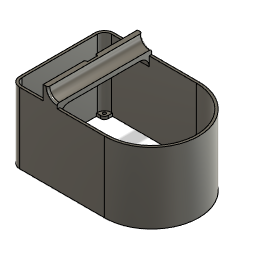
planter base v6 (Autodesk Fusion 360 design; units mm, degrees)
Autodesk Fusion 360 part; units mm, degrees
sketch "スケッチ1" plane through (0, 0, 0) normal (0, 1, 0) x (1, 0, 0)
  line L0 (0, -146.8474) -> (0, 139.3157) construction
  line L1 (0, -50) -> (-90, -50)
  line L2 (0, 50) -> (-90, 50)
  line L3 (-100, -40) -> (-100, 40)
  arc A0 (-100, -40) -> (-90, -50) centre (-90, -40) ccw
  arc A1 (-90, 50) -> (-100, 40) centre (-90, 40) ccw
  line L4 (0, -47.5) -> (-90, -47.5)
  arc A2 (-97.5, -40) -> (-90, -47.5) centre (-90, -40) ccw
  line L5 (-97.5, -40) -> (-97.5, 40)
  arc A3 (-90, 47.5) -> (-97.5, 40) centre (-90, 40) ccw
  line L6 (0, 47.5) -> (-90, 47.5)
  arc A4 (0, -47.5) -> (0, 47.5) centre (0, 0) ccw
  arc A5 (0, -50) -> (0, 50) centre (0, 0) ccw
  line L7 (-65, -50) -> (-65, 50)
  line L8 (-60, -50) -> (-60, 50)
  line L9 (-50, -50) -> (-50, 50)
  line L10 (-55.4985, -5.25) -> (-69.5015, -5.25) construction
  line L11 (-56.3526, 5.25) -> (-68.6474, 5.25) construction
  line L12 (-56.8132, 6.25) -> (-69.108, 6.25) construction
  line L13 (-56.8132, -6.25) -> (-69.108, -6.25) construction
  line L14 (-62.5, -5.25) -> (-62.5, 5.25)
  line L15 (-62.5, -5.25) -> (-65, -6.25)
  line L16 (-62.5, 5.25) -> (-65, 6.25)
  line L17 (0, -40) -> (0, -47.5)
  line L18 (0, 40) -> (0, 47.5)
  arc A6 (0, -40) -> (0, 40) centre (0, 0) ccw
  line L19 (150.4172, 0) -> (40, 0) construction
  line L20 (0, 0) -> (-159.0811, 0) construction
  line L21 (-89, 47.5) -> (-89, -47.5) construction
  line L22 (-8, -47.5) -> (-8, -44)
  line L23 (-4, -40) -> (0, -40)
  line L24 (-8, 47.5) -> (-8, 44)
  line L25 (-4, 40) -> (0, 40)
  arc A7 (-4, -40) -> (-8, -44) centre (-4, -44) ccw
  arc A8 (-8, 44) -> (-4, 40) centre (-4, 44) ccw
  circle A9 centre (-4, -44) radius 1.6
  circle A10 centre (-4, 44) radius 1.6
  circle A11 centre (-93, -43) radius 1.6
  circle A12 centre (-93, 43) radius 1.6
  circle A13 centre (44, 0) radius 1.6
  line L26 (-97.5, 39) -> (-93, 39)
  line L27 (-97.5, -39) -> (-93, -39)
  line L28 (-89, -43) -> (-89, -47.5)
  line L29 (-89, 43) -> (-89, 47.5)
  arc A14 (-89, -43) -> (-93, -39) centre (-93, -43) ccw
  arc A15 (-93, 39) -> (-89, 43) centre (-93, 43) ccw
  dimension "d1" = 100
  dimension "d2" = 95
  dimension "d3" = 100
  dimension "d4" = 10
  dimension "d5" = 10
  dimension "d6" = 2.5
  dimension "d7" = 5
  dimension "d8" = 60
  dimension "d9" = 10
  dimension "d10" = 5.25
  dimension "d11" = 1
  dimension "d12" = 10.5
  dimension "d13" = 12.5
  dimension "d14" = 2.5
  dimension "d34" = 80
  dimension "d35" = 11
  dimension "d36" = 8
  dimension "d37" = 8
  dimension "d38" = 4
  dimension "d39" = 3.2
  dimension "d40" = 3.2
  dimension "d41" = 3.2
  dimension "d42" = 3.2
  dimension "d43" = 3.2
  dimension "d44" = 44
  dimension "d52" = 40
  dimension "d53" = 30
  dimension "d54" = 7
  dimension "d55" = 7
  dimension "d56" = 7
  dimension "d57" = 7
  dimension "d58" = 6
  dimension "d59" = 4
  dimension "d60" = 6
  dimension "d61" = 4
  dimension "d62" = 11
  dimension "d63" = 11
  dimension "d64" = 4
  dimension "d65" = 4
  constraint horizontal L19
  constraint perpendicular L0 L19
  constraint coincident A4.centre A5.centre
  constraint concentric A4 A5
  constraint coincident L0 L1.start
  constraint tangent L1 A5
  constraint coincident L0 L2.start
  constraint tangent L2 A5
  constraint perpendicular L0 L2
  constraint perpendicular L1 L3
  constraint tangent L1 A0
  constraint tangent L3 A0
  constraint tangent L3 A1
  constraint tangent L2 A1
  constraint coincident L1 L7.start
  constraint coincident L2 L7.end
  constraint perpendicular L2 L7
  constraint coincident L1 L8.start
  constraint coincident L2 L8.end
  constraint perpendicular L2 L8
  constraint coincident L1 L9.start
  constraint coincident L2 L9.end
  constraint perpendicular L2 L9
  constraint perpendicular L7 L10
  constraint perpendicular L7 L11
  constraint perpendicular L7 L12
  constraint perpendicular L7 L13
  constraint midpoint L10 L14.start
  constraint midpoint L11 L14.end
  constraint parallel L7 L14
  constraint coincident L13 L15.end
  constraint coincident L7 L15.end
  constraint coincident L12 L16.end
  constraint coincident L7 L16.end
  constraint concentric A4 A6
  constraint coincident L0 L17.start
  constraint perpendicular L4 L17
  constraint coincident L0 L18.start
  constraint perpendicular L6 L18
  constraint coincident A6 L19.end
  constraint collinear L19 L20
  constraint coincident L6 L21.start
  constraint coincident L4 L21.end
  constraint perpendicular L4 L21
  constraint coincident L4 L22.start
  constraint perpendicular L4 L22
  constraint tangent A6 L23
  constraint coincident L6 L24.start
  constraint perpendicular L23 L24
  constraint tangent A6 L25
  constraint tangent L22 A7
  constraint tangent L23 A7
  constraint tangent L24 A8
  constraint tangent L25 A8
  constraint equal A7 A8
  constraint coincident L19 A13.centre
  constraint perpendicular L21 L26
  constraint coincident L5 L27.start
  constraint perpendicular L21 L27
  constraint coincident L5 L26.start
  constraint tangent L27 A14
  constraint tangent L28 A14
  constraint collinear L21 L28
  constraint tangent L26 A15
  constraint tangent L29 A15
  constraint collinear L21 L29
  measures "d1" diameter of A5
  measures "d2" diameter of A4
  measures "d3" distance of L0 L3
  measures "d4" radius of A0
  measures "d5" radius of A1
  measures "d7" distance of L7 L8
  measures "d8" distance of L0 L8
  measures "d9" distance of L8 L9
  measures "d10" distance of L10 L19
  measures "d11" distance of L10 L13
  measures "d12" distance of L10 L11
  measures "d13" distance of L12 L13
  measures "d14" distance of L7 L14
  measures "d34" diameter of A6
  measures "d35" distance of L3 L21
  measures "d36" distance of L18 L24
  measures "d37" distance of L0 L22
  measures "d38" radius of A7
  measures "d39" diameter of A9
  measures "d40" diameter of A10
  measures "d41" diameter of A11
  measures "d42" diameter of A12
  measures "d43" diameter of A13
  measures "d44" distance of A4.centre A13.centre
  measures "d52" distance of L3 L8
  measures "d53" distance of A3.start L8
  measures "d54" distance of L1 A11.centre
  measures "d55" distance of L3 A11.centre
  measures "d56" distance of L3 A12.centre
  measures "d57" distance of L2 A12.centre
  measures "d58" distance of L1 A7.centre
  measures "d59" distance of L0 A7.centre
  measures "d60" distance of L2 A8.centre
  measures "d61" distance of L0 A8.centre
  measures "d62" distance of L2 L26
  measures "d63" distance of L1 L27
  measures "d64" radius of A14
  measures "d65" radius of A15
extrude "押し出し1" add sketch "スケッチ1" along normal blind 15 contours L1 L4 L7 L8 | L4 L6 L7 L8 L14 L15 L16 | L2 L6 L7 L8
extrude "押し出し2" add sketch "スケッチ1" along normal blind 5 contours L1 L4 L8 L9 | L4 L6 L8 L9 | L2 L6 L8 L9
fillet "フィレット1" radius 10 1 edges at (-60, 5, 0)
extrude "押し出し3" add sketch "スケッチ1" against normal blind 75 contours L1 L2 L4 L6 A4 A5 L9 | L1 L4 L8 L9 | L1 L4 L7 L8 | L2 L6 L8 L9 | L1 L2 L3 A0 A1 L4 A2 L5 A3 L6 L7 | L2 L6 L7 L8
fillet "フィレット2" radius 10 2 edges at (-57.5, 0, 47.5) (-57.5, 0, -47.5)
sketch "スケッチ2" plane through (-65, 0, 0) normal (-1, 0, 0) x (0, 0, 1)
  line L0 (-37.5, 0) -> (-6.25, 0)
  line L1 (-6.25, 0) -> (-6.25, 15)
  line L2 (-6.25, 15) -> (-50, 15)
  line L3 (-50, 15) -> (-50, 0)
  line L4 (-50, 0) -> (-47.5, 0)
  line L5 (-47.5, 0) -> (-47.5, -10)
  arc A0 (-37.5, 0) -> (-47.5, -10) centre (-37.5, -10) ccw
  line L6 (-50, 0) -> (50, 0) construction
  line L7 (50, 0) -> (50, 15) construction
  line L8 (50, 15) -> (-50, 15) construction
  line L9 (-50, 15) -> (-50, 0) construction
  line L10 (40, 0) -> (-40, 0) construction
  line L11 (-60.3557, 7.5) -> (64.0451, 7.5) construction
  line L12 (-30, 22.008) -> (-30, -9.3595) construction
  line L13 (30, 22.008) -> (30, -9.3595) construction
  circle A1 centre (-30, 7.5) radius 1.3
  circle A2 centre (30, 7.5) radius 1.3
  dimension "d25" = 100
  dimension "d26" = 15
  dimension "d27" = 20
  dimension "d28" = 20
  dimension "d29" = 7.5
  dimension "d30" = 2.6
  dimension "d31" = 2.6
  constraint horizontal L6
  constraint vertical L7
  constraint horizontal L8
  constraint vertical L9
  constraint coincident L3.end L4.start
  constraint perpendicular L7 L11
  constraint perpendicular L6 L12
  constraint perpendicular L6 L13
  constraint coincident L11 A1.centre
  constraint coincident L12 A1.centre
  constraint coincident L13 A2.centre
  constraint coincident L11 A2.centre
  measures "d25" distance of L7 L9
  measures "d26" distance of L8 L10
  measures "d27" distance of L9 L12
  measures "d28" distance of L7 L13
  measures "d29" distance of L10 L11
  measures "d30" diameter of A1
  measures "d31" diameter of A2
extrude "押し出し4" cut sketch "スケッチ2" against normal blind 5 contours A1 | A2
extrude "押し出し5" add sketch "スケッチ1" along normal blind 3 from surface at -75 contours L4 L17 L22 L23 A7 | A4 L17 L18 A6 | L6 L18 L24 L25 A8 | L4 A2 L5 L27 L28 A14 | L5 A3 L6 L26 L29 A15
fillet "フィレット4" radius 2 2 edges at (-57.0711, 7.9289, 50) (-57.0711, 7.9289, -50)
